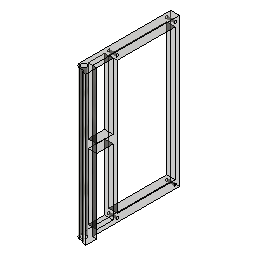
FRW (Autodesk Fusion 360 archive; units mm, degrees)
design "90 deg flap"
Autodesk Fusion 360 part; units mm, degrees
sketch "Sketch1" plane through (0, 0, 0) normal (0, 0, 1) x (1, 0, 0)
  circle A0 centre (0, 0) radius 3.25
  line L0 (0, 0) -> (0, -3.25)
  line L1 (0, -3.25) -> (0, -5.25)
  line L2 (0, -6.25) -> (0, -28.75)
  circle A1 centre (0, -28.75) radius 22.5
  circle A2 centre (0, 0) radius 5.25
  line L3 (0, -5.25) -> (5.25, -5.25)
  line L4 (5.25, -5.25) -> (5.25, -6.8711)
  line L5 (10.25, -5.25) -> (10.25, -8.7203)
  line L6 (10.25, -5.25) -> (10.25, 5.25)
  line L7 (10.25, 5.25) -> (5.25, 5.25)
  line L8 (0, 0) -> (0, 110)
  line L9 (5.25, 5.25) -> (5.25, 110)
  line L10 (0, 110) -> (5.25, 110)
  line L11 (0, 110) -> (-5.25, 110)
  line L12 (-5.25, 110) -> (-5.25, 0)
  dimension "d1" = 6.5
  dimension "d2" = 2
  dimension "d3" = 1
  dimension "d4" = 22.5
  dimension "d5" = 5.25
  dimension "d6" = 5
  dimension "d8" = 5
  dimension "d9" = 110
  dimension "d10" = 104.75
  dimension "d11" = 5.25
  constraint coincident A0.centre L0.start
  constraint coincident A0 L0.end
  constraint vertical L0
  constraint parallel L0 L1
  constraint coincident L2.end A1.centre
  constraint coincident L2.start A1
  constraint coincident L1.end A2
  constraint perpendicular L1 L3
  constraint coincident A1 L4.end
  constraint perpendicular L3 L4
  constraint coincident A1 L5.end
  constraint perpendicular L6 L7
  constraint parallel L0 L8
  constraint perpendicular L7 L9
  constraint perpendicular L8 L11
  constraint coincident A2 L12.end
  constraint tangent A2 L12
  measures "d1" diameter of A0
  measures "d2" distance of L0.end L1.end
  measures "d3" distance of L1.end L2.start
  measures "d4" distance of L2.start L2.end
  measures "d5" distance of L1.end L3.end
  measures "d6" distance of L3.end L5.start
  measures "d8" distance of L6.end L7.end
  measures "d9" distance of A0.centre L8.end
  measures "d10" distance of L7.end L9.end
  measures "d11" distance of L8.end L11.end
extrude "Extrude1" add sketch "Sketch1" along normal blind 179 contours A0 L1 A2 L8 | A0 L1 A2 L8 | A1 A2 L3 L4 L5 L6 L7 L8 L9 L10 | A2 L8 L11 L12 makes body 1
sketch "Sketch2" plane through (-5.25, 0, 0) normal (-1, 0, 0) x (0, -1, 0)
  line L0 (-110, 0) -> (-110, 179)
  line L1 (-5.25, 0) -> (-5.25, 179)
  line L2 (-110, 89.5) -> (-5.25, 89.5)
  line L3 (-110, 89.5) -> (-70, 89.5)
  line L4 (-35, 169.5) -> (-105, 169.5)
  line L5 (-105, 169.5) -> (-105, 9.5)
  line L6 (-105, 9.5) -> (-35, 9.5)
  line L7 (-35, 9.5) -> (-35, 169.5)
  line L8 (-35, 169.5) -> (-105, 9.5) construction
  line L9 (-105, 169.5) -> (-35, 9.5) construction
  line L10 (-105, 174.5) -> (-35, 174.5)
  line L11 (-35, 174.5) -> (-35, 4.5)
  line L12 (-35, 4.5) -> (-105, 4.5)
  line L13 (-105, 4.5) -> (-105, 174.5)
  line L14 (-105, 174.5) -> (-35, 4.5) construction
  line L15 (-35, 174.5) -> (-105, 4.5) construction
  circle A0 centre (-105, 174.5) radius 1.5
  circle A1 centre (-35, 174.5) radius 1.5
  circle A2 centre (-105, 4.5) radius 1.5
  circle A3 centre (-35, 4.5) radius 1.5
  point P0 (-70, 89.5)
  point P1 (-70, 89.5)
  dimension "d14" = 40
  dimension "d15" = 70
  dimension "d16" = 160
  dimension "d23" = 70
  dimension "d24" = 170
  dimension "d25" = 3
  dimension "d26" = 3
  dimension "d27" = 3
  dimension "d28" = 3
  constraint midpoint L0 L2.start
  constraint midpoint L1 L2.end
  constraint perpendicular L0 L3
  constraint horizontal L4
  constraint perpendicular L4 L5
  constraint parallel L4 L6
  constraint parallel L5 L7
  constraint coincident L8 P1
  constraint coincident L9 P1
  constraint coincident P1 P0
  constraint horizontal L10
  constraint perpendicular L10 L11
  constraint parallel L10 L12
  constraint parallel L11 L13
  constraint coincident L14 P1
  constraint coincident L15 P1
  constraint coincident L10.start L13.end
  constraint coincident L10.end L11.start
  constraint coincident L12.end L13.start
  constraint coincident L11.end L12.start
  measures "d14" distance of L2.start P1
  measures "d15" distance of L5.end L6.end
  measures "d16" distance of L4.end L5.end
  measures "d23" distance of L11.end L12.end
  measures "d24" distance of L10.end L11.end
  measures "d25" diameter of A0
  measures "d26" diameter of A1
  measures "d27" diameter of A2
  measures "d28" diameter of A3
extrude "Extrude2" cut sketch "Sketch2" against normal blind 10.5 contours L2 L3 L4 L5 L7 L11 L13 | L2 L3 L5 L6 L7 L11 L13 | L10 L13 A0 | L10 L13 A0 | L12 L13 A2 | L12 L13 A2 | L10 L11 A1 | L10 L11 A1 | L11 L12 A3 | L11 L12 A3 bodies 1
sketch "Sketch3" plane through (-5.25, 0, 0) normal (-1, 0, 0) x (0, -1, 0)
  line L0 (-35, 9.5) -> (-35, 169.5)
  line L1 (-5.25, 0) -> (-5.25, 179)
  line L2 (-35, 89.5) -> (-5.25, 89.5)
  line L3 (-110, 0) -> (0, 0)
  line L4 (-20.125, 89.5) -> (-20.125, 0)
  line L5 (-110, 179) -> (0, 179)
  line L6 (-20.125, 89.5) -> (-20.125, 179)
  line L7 (-20.125, 89.5) -> (-20.125, 0)
  line L8 (-10.25, 84.5) -> (-30, 84.5)
  line L9 (-30, 84.5) -> (-30, 5)
  line L10 (-30, 5) -> (-10.25, 5)
  line L11 (-10.25, 5) -> (-10.25, 84.5)
  line L12 (-10.25, 84.5) -> (-30, 5) construction
  line L13 (-30, 84.5) -> (-10.25, 5) construction
  line L14 (-10.25, 94.5) -> (-30, 94.5)
  line L15 (-30, 94.5) -> (-30, 174)
  line L16 (-10.25, 174) -> (-10.25, 94.5)
  line L17 (-30, 174) -> (-10.25, 174)
  point P0 (-20.125, 44.75)
  point P1 (-20.125, 44.75)
  dimension "d19" = 19.75
  dimension "d20" = 79.5
  constraint midpoint L0 L2.start
  constraint midpoint L1 L2.end
  constraint midpoint L2 L4.start
  constraint coincident L3 L4.end
  constraint perpendicular L2 L4
  constraint coincident L5 L6.end
  constraint perpendicular L2 L6
  constraint midpoint L7 P1
  constraint horizontal L8
  constraint perpendicular L8 L9
  constraint parallel L8 L10
  constraint parallel L9 L11
  constraint coincident L12 P1
  constraint coincident L13 P1
  constraint coincident P1 P0
  constraint symmetric L2 L8.start L14.start
  constraint symmetric L2 L8.end L14.end
  constraint symmetric L2 L9.end L15.end
  constraint symmetric L2 L10.end L16.start
  measures "d19" distance of L9.end L10.end
  measures "d20" distance of L8.end L9.end
extrude "Extrude3" cut sketch "Sketch3" against normal blind 25 contours L4 L7 L8 L9 L10 | L4 L7 L8 L10 L11 | L6 L14 L15 L17 | L6 L14 L16 L17 bodies 1
sketch "Sketch4" plane through (-5.25, 0, 0) normal (-1, 0, 0) x (0, -1, 0)
copy_body "Body->Comp1" bodies 1 removing the originals makes body 2 in component "Component"
component "Component" placed x (1, 0, 0) y (0, 1, 0) z (0, 0, 1) at (0, 0, 0)
equation "d5 = ( 10.5 / 2 ) * 1 mm"
equation "d10 = 110 mm - ( 10.5 / 2 ) * 1 mm"
equation "d16 = 180 mm - ( 10 * 2 ) * 1 mm"
equation "d19 = 29.75 mm - 10 mm"
equation "d20 = 89.5 mm - ( 5 * 2 ) * 1 mm"
equation "d23 = 80 mm - 10 mm"

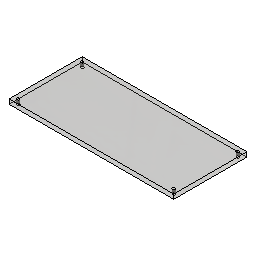
design "Simple Flat Bucket"
Autodesk Fusion 360 part; units mm, degrees
sketch "Sketch1" plane through (0, 0, 0) normal (0, 0, 1) x (1, 0, 0)
  line L0 (90, -40) -> (-90, -40)
  line L1 (-90, -40) -> (-90, 40)
  line L2 (-90, 40) -> (90, 40)
  line L3 (90, 40) -> (90, -40)
  line L4 (90, -40) -> (-90, 40) construction
  line L5 (-90, -40) -> (90, 40) construction
  line L6 (-85, -35) -> (85, 35) construction
  line L7 (85, -35) -> (-85, 35) construction
  circle A0 centre (-85, 35) radius 1.5
  circle A1 centre (-85, -35) radius 1.5
  circle A2 centre (85, 35) radius 1.5
  circle A3 centre (85, -35) radius 1.5
  dimension "d1" = 180
  dimension "d2" = 80
  dimension "d3" = 170
  dimension "d4" = 70
  dimension "d5" = 3
  dimension "d6" = 3
  dimension "d7" = 3
  dimension "d8" = 3
  constraint horizontal L0
  constraint perpendicular L0 L1
  constraint parallel L0 L2
  constraint parallel L1 L3
  constraint coincident L4 origin
  constraint coincident L5 origin
  constraint coincident L6 origin
  constraint coincident L7 origin
  constraint coincident L7.end A0.centre
  constraint coincident L6.start A1.centre
  constraint coincident L6.end A2.centre
  constraint coincident L7.start A3.centre
  measures "d1" distance of L1.end L2.end
  measures "d2" distance of L0.end L1.end
  measures "d3" distance of L6.end L7.end
  measures "d4" distance of L7.start L6.end
  measures "d5" diameter of A0
  measures "d6" diameter of A1
  measures "d7" diameter of A2
  measures "d8" diameter of A3
extrude "Extrude1" add sketch "Sketch1" along normal blind 5 makes body 1
copy_body "Body->Comp1" bodies 1 removing the originals makes body 2 in component "Simple flat bucket"
component "Simple flat bucket" placed x (1, 0, 0) y (0, 1, 0) z (0, 0, 1) at (0, 0, 0)

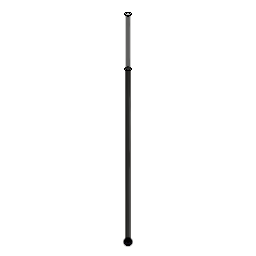
design "Aluminum 4mm 6mm bar"
Autodesk Fusion 360 part; units mm, degrees
sketch "Aluminum 4mm-6mm" plane through (0, 0, 0) normal (0, 0, 1) x (1, 0, 0)
  circle A0 centre (0, 0) radius 2
  circle A1 centre (0, 0) radius 3
  dimension "d1" = 4
  dimension "d2" = 6
  constraint coincident A0.centre A1.centre
  measures "d1" diameter of A0
  measures "d2" diameter of A1
extrude "Extrude1" add sketch "Aluminum 4mm-6mm" along normal blind 190 makes body 1
copy_body "Body->Comp1" bodies 1 removing the originals makes body 2 in component "190mm aluminum 4-6 bar"
extrude "Extrude2" add sketch "Aluminum 4mm-6mm" along normal blind 250 separate body makes body 3
copy_body "Body->Comp2" bodies 3 removing the originals makes body 4 in component "250mm aluminum 4-6 bar"
component "190mm aluminum 4-6 bar" placed x (1, 0, 0) y (0, 1, 0) z (0, 0, 1) at (0, 0, 0)
component "250mm aluminum 4-6 bar" placed x (1, 0, 0) y (0, 1, 0) z (0, 0, 1) at (0, 0, 0)
